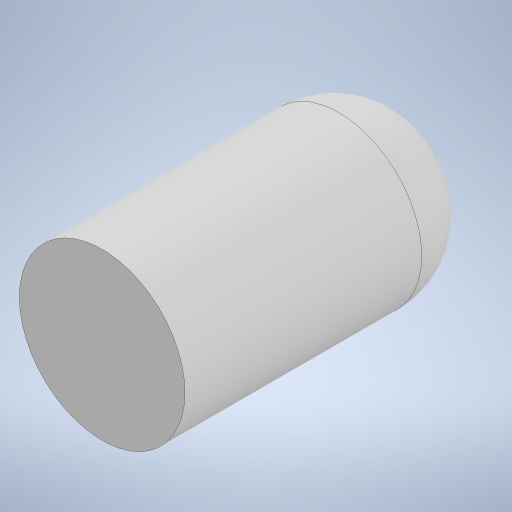
# Autodesk Inventor part: ex_tank_H
Saved by Autodesk Inventor 2024 (Build 280153000, 153)
## iProperties
Created: 2023-06-07
Part Number: ex_tank_H
Material: Generic
Document SubType Name: Modeling
Designer: tamiz
Density: 1 g/cm^3
Appearance: Default
Author: tamiz
Autodesk Inventor part; units mm, degrees
ref_plane "YZ Plane" through (0, 0, 0) normal (1, 0, 0) x (0, 1, 0)
ref_plane "XZ Plane" through (0, 0, 0) normal (0, 1, 0) x (-1, 0, 0)
ref_plane "XY Plane" through (0, 0, 0) normal (0, 0, 1) x (1, 0, 0)
sketch "Sketch1" plane through (0, 0, 0) normal (0, 0, 1) x (1, 0, 0)
  circle A0 centre (0, 0) radius 5334
  dimension "d0" = 10668
  constraints: 1 centre point, 1 coincident
  measures "d0" diameter of A0
extrude "Extrusion1" add sketch "Sketch1" against normal blind 19812
sketch "Sketch2" plane through (0, 0, 0) normal (0, 0, 1) x (1, 0, 0)
  circle A0 centre (0, 0) radius 4876.8
  constraints: 1 centre point, 1 coincident
fillet "Fillet1" radius 4572 1 edges at (-5334, 0, -19812)
sketch "Sketch3" plane through (0, 0, 0) normal (1, 0, 0) x (0, 1, 0)
  line L0 (0, -15240) -> (0, -19354.8)
  line L1 (0, -15240) -> (4876.8, -15240)
  arc A0 (762, -19354.8) -> (4876.8, -15240) centre (762, -15240) ccw
  line L2 (762, -19354.8) -> (0, -19354.8)
  point P0 (0, 0)
  constraints: 6 end point, 2 point on circle, 1 centre point, 1 horizontal, 1 vertical
revolve "Revolution1" cut sketch "Sketch3" angle 360 about axis through (0, 0, -15240) along (0, 0, -1)
extrude "Extrusion2" cut sketch "Sketch2" against normal blind 15240
sketch "Sketch4" plane through (0, 0, 0) normal (0, 0, 1) x (1, 0, 0)
  circle A0 centre (0, 0) radius 5334
  constraints: 1 centre point, 1 coincident
extrude "Extrusion3" add sketch "Sketch4" against normal blind 457.2
body "Solid1"
